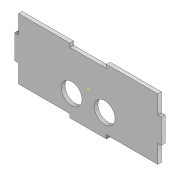
# Autodesk Inventor part: 본체 겉면 레이저 앞판 수정
Saved by Autodesk Inventor 2020 (Build 240168000, 168)
## iProperties
Created: 2022-08-25
Part Number: 본체 겉면 레이저 앞판 수정
Material: 일반
Document SubType Name: Modeling
Designer: 박연호
Density: 1 g/cm^3
Appearance: 기본값
Author: 박연호
Autodesk Inventor part; units mm, degrees
ref_plane "YZ Plane" through (0, 0, 0) normal (1, 0, 0) x (0, 1, 0)
ref_plane "XZ Plane" through (0, 0, 0) normal (0, 1, 0) x (-1, 0, 0)
ref_plane "XY Plane" through (0, 0, 0) normal (0, 0, 1) x (1, 0, 0)
sketch "스케치1" plane through (0, 0, 0) normal (0, 0, 1) x (1, 0, 0)
  line L0 (-60, -25) -> (60, -25)
  line L1 (60, -25) -> (60, 25)
  line L2 (60, 25) -> (-60, 25)
  line L3 (-60, 25) -> (-60, -25)
  line L4 (-60, -25) -> (60, 25) construction
  line L5 (60, -25) -> (-60, 25) construction
  point P0 (0, 0)
  dimension "d0" = 120
  dimension "d1" = 50
  constraints: 12 end point, 2 midpoint, 2 parallel, 1 horizontal, 1 perpendicular
  measures "d0" distance of L2.end L1.end
  measures "d1" distance of L0.end L1.end
extrude "돌출1" add sketch "스케치1" along normal blind 3
sketch "스케치2" plane through (0, 0, 3) normal (0, 0, 1) x (1, 0, 0)
  line L0 (60, 25) -> (-60, 25) projected
  line L1 (60, 25) -> (57, 25)
  line L2 (57, 25) -> (57, 10)
  line L3 (57, 10) -> (60, 10)
  line L4 (60, 10) -> (60, 25)
  line L5 (-60, 0) -> (60, 0)
  line L6 (60, -25) -> (60, 25) projected
  line L7 (0, 25) -> (0, -25)
  line L8 (-60, -25) -> (60, -25) projected
  line L9 (60, -25) -> (57, -25)
  line L10 (57, -25) -> (57, -10)
  line L11 (57, -10) -> (60, -10)
  line L12 (60, -10) -> (60, -25)
  line L13 (-60, 25) -> (-57, 25)
  line L14 (-57, 25) -> (-57, 10)
  line L15 (-57, 10) -> (-60, 10)
  line L16 (-60, 10) -> (-60, 25)
  line L17 (-60, -25) -> (-57, -25)
  line L18 (-57, -25) -> (-57, -10)
  line L19 (-57, -10) -> (-60, -10)
  line L20 (-60, -10) -> (-60, -25)
  point P0 (0, 0)
  dimension "d4" = 3
  dimension "d5" = 15
  constraints: 36 end point, 9 symmetric about line, 3 midpoint, 2 parallel, 1 horizontal, 1 perpendicular
  measures "d4" distance between parallel lines of L4 L2
  measures "d5" distance of L3.end L0.start
extrude "돌출2" cut sketch "스케치2" against normal through all contours L4 L3 L2 L0 | L8 L20 L19 L18 | L14 L15 L16 L0 | L6 L8 L10 L11
sketch "스케치3" plane through (0, 0, 3) normal (0, 0, 1) x (1, 0, 0)
  line L0 (-15, 22) -> (15, 22)
  line L1 (15, 22) -> (15, 28)
  line L2 (15, 28) -> (-15, 28)
  line L3 (-15, 28) -> (-15, 22)
  line L4 (57, 25) -> (-57, 25) projected
  line L5 (-15, 22) -> (15, 28) construction
  line L6 (15, 22) -> (-15, 28) construction
  point P0 (0, 0)
  point P1 (0, 25)
  point P2 (15, 25)
  point P3 (-15, 25)
  dimension "d8" = 30
  dimension "d9" = 3
  constraints: 12 end point, 3 midpoint, 2 parallel, 1 horizontal, 1 perpendicular
  measures "d8" distance of L2.end L1.end
  measures "d9" distance between parallel lines of L0 L4
extrude "돌출3" cut sketch "스케치3" against normal through all contours L3 L4 L1 L0
sketch "스케치4" plane through (0, 0, 3) normal (0, 0, 1) x (1, 0, 0)
  line L0 (-15, -28) -> (15, -28)
  line L1 (15, -28) -> (15, -22)
  line L2 (15, -22) -> (-15, -22)
  line L3 (-15, -22) -> (-15, -28)
  line L4 (-57, -25) -> (57, -25) projected
  line L5 (-15, -28) -> (15, -22) construction
  line L6 (15, -28) -> (-15, -22) construction
  point P0 (0, 0)
  point P1 (0, -25)
  point P2 (15, -25)
  point P3 (-15, -25)
  dimension "d12" = 3
  dimension "d13" = 30
  constraints: 12 end point, 3 midpoint, 2 parallel, 1 horizontal, 1 perpendicular
  measures "d12" distance between parallel lines of L0 L4
  measures "d13" distance of L1.end L2.end
extrude "돌출4" add sketch "스케치4" against normal blind 3 contours L3 L4 L1 L0
sketch "스케치5" plane through (0, 0, 3) normal (0, 0, 1) x (1, 0, 0)
  circle A0 centre (-13.5, -10) radius 8.5
  circle A1 centre (13.5, -10) radius 8.5
  line L0 (15, -25) -> (57, -25) projected
  line L1 (-57, -25) -> (-15, -25) projected
  line L2 (60, -10) -> (60, 10) projected
  point P0 (0, 0)
  dimension "d16" = 27
  dimension "d18" = 17
  dimension "d19" = 17
  dimension "d22" = 15
  dimension "d23" = 15
  dimension "d24" = 46.5
  constraints: 2 centre point
  measures "d16" distance of A1.centre A0.centre
  measures "d18" diameter of A0
  measures "d19" diameter of A1
  measures "d22" distance from line of L0 A1.centre
  measures "d23" distance from line of L1 A0.centre
  measures "d24" distance from line of L2 A1.centre
extrude "돌출5" cut sketch "스케치5" against normal through all
sketch "스케치6" plane through (0, 0, 3) normal (0, 0, 1) x (1, 0, 0)
  point P0 (0, 0)
sketch "스케치7" plane through (0, 0, 3) normal (0, 0, 1) x (1, 0, 0)
  point P0 (0, 0)
